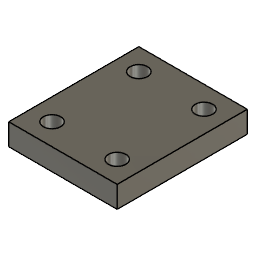
_HTD 3M Belt Clamp 2 pt 2.d0539dd2-3fbc-4beb-923a-612518bf1b36 (Autodesk Fusion 360 design; units mm, degrees)
Autodesk Fusion 360 part; units mm, degrees
sketch "Sketch1" plane through (0, 0, 0) normal (0, 0, 1) x (1, 0, 0)
  line L0 (0, 0) -> (25, 0)
  line L1 (25, 0) -> (25, 30)
  line L2 (25, 30) -> (0, 30)
  line L3 (0, 30) -> (0, 0)
  dimension "d1" = 25
  dimension "d2" = 30
  constraint horizontal L0
  constraint vertical L1
  constraint horizontal L2
  constraint vertical L3
  constraint coincident L0.start L3.end
  measures "d1" distance of L0.start L0.end
  measures "d2" distance of L0.start L2.end
sketch "Sketch2" plane through (0, 0, 0) normal (0, -1, 0) x (1, 0, 0)
  line L0 (0, 0) -> (25, 0)
  line L1 (25, 0) -> (25, 4)
  line L2 (25, 4) -> (0, 4)
  line L3 (0, 4) -> (0, 0)
  line L4 (25, 2.86) -> (0, 2.86)
  line L5 (0.89, 4) -> (1.1955, 2.86)
  line L6 (2.3645, 2.86) -> (2.67, 4)
  line L7 (3.89, 4) -> (4.1955, 2.86)
  line L8 (5.3645, 2.86) -> (5.67, 4)
  line L9 (6.89, 4) -> (7.1955, 2.86)
  line L10 (8.3645, 2.86) -> (8.67, 4)
  line L11 (9.89, 4) -> (10.1955, 2.86)
  line L12 (11.3645, 2.86) -> (11.67, 4)
  line L13 (12.89, 4) -> (13.1955, 2.86)
  line L14 (14.3645, 2.86) -> (14.67, 4)
  line L15 (15.89, 4) -> (16.1955, 2.86)
  line L16 (17.3645, 2.86) -> (17.67, 4)
  line L17 (18.89, 4) -> (19.1955, 2.86)
  line L18 (20.3645, 2.86) -> (20.67, 4)
  line L19 (21.89, 4) -> (22.1955, 2.86)
  line L20 (23.3645, 2.86) -> (23.67, 4)
  dimension "d5" = 1.14
  dimension "d7" = 1.78
  dimension "d8" = 0.89
  dimension "d11" = 3
  dimension "d12" = 0
  dimension "d15" = 30
  constraint coincident L1 L4.start
  constraint coincident L3 L4.end
  constraint perpendicular L3 L4
  constraint coincident L2 L5.start
  constraint coincident L4 L5.end
  constraint coincident L4 L6.start
  constraint coincident L2 L6.end
  constraint equal L5 L6
  measures "d5" distance of L2 L4
  measures "d7" distance of L5.start L6.end
  measures "d8" distance of L2.end L5.start
  measures "d15" angle of L5 L6
sketch "Sketch3" plane through (0, 0, 0) normal (0, 0, -1) x (1, 0, 0)
  line L0 (0, 0) -> (0, -30)
  line L1 (0, -30) -> (25, -30)
  line L2 (25, -30) -> (25, 0)
  line L3 (25, 0) -> (0, 0)
  line L4 (20, -25) -> (5, -25) construction
  line L5 (5, -25) -> (5, -5) construction
  line L6 (5, -5) -> (20, -5) construction
  line L7 (20, -5) -> (20, -25) construction
  circle A0 centre (20, -25) radius 2
  circle A1 centre (5, -25) radius 2
  circle A2 centre (20, -5) radius 2
  circle A3 centre (5, -5) radius 2
  point P0 (12.5, -25)
  point P1 (5, -15)
  point P2 (0, -15)
  point P3 (12.5, -30)
  dimension "d16" = 15
  dimension "d17" = 20
  dimension "d18" = 4
  dimension "d19" = 4
  constraint horizontal L4
  constraint vertical L5
  constraint horizontal L6
  constraint vertical L7
  constraint midpoint L4 P0
  constraint midpoint L5 P1
  constraint midpoint L0 P2
  constraint horizontal P1 P2
  constraint midpoint L1 P3
  constraint vertical P0 P3
  constraint coincident L4.start L7.end
  constraint coincident L4.end L5.start
  constraint coincident L6.end L7.start
  constraint coincident L5.end L6.start
  constraint equal A2 A3
  constraint equal A0 A2
  measures "d16" distance of L4.start L4.end
  measures "d17" distance of L4.end L5.end
  measures "d18" diameter of A0
  measures "d19" diameter of A1
mirror "Mirror1" [no effect]
extrude "Extrude4" add sketch "Sketch3" along normal blind 5
equation "d8 = ( 1.78 / 2 ) * 1 mm"
